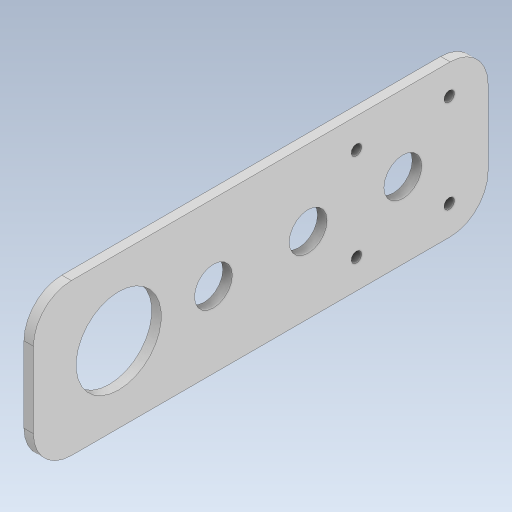
# Autodesk Inventor part: Housing
Saved by Autodesk Inventor 2023 (Build 270158000, 158)
## iProperties
Created: 2023-01-21
Part Number: Housing
Material: Generic
Document SubType Name: Modeling
Designer: Dave
Density: 1 g/cm^3
Appearance: Default
Author: Dave
Autodesk Inventor part; units mm, degrees
ref_plane "YZ Plane" through (0, 0, 0) normal (1, 0, 0) x (0, 1, 0)
ref_plane "XZ Plane" through (0, 0, 0) normal (0, 1, 0) x (-1, 0, 0)
ref_plane "XY Plane" through (0, 0, 0) normal (0, 0, 1) x (1, 0, 0)
sketch "Sketch1" plane through (0, 0, 0) normal (1, 0, 0) x (0, 1, 0)
  line L0 (12.7, 0) -> (38.1, 0)
  line L1 (50.8, -12.7) -> (50.8, -139.7)
  line L2 (38.1, -152.4) -> (12.7, -152.4)
  line L3 (0, -139.7) -> (0, -12.7)
  arc A0 (50.8, -12.7) -> (38.1, 0) centre (38.1, -12.7) ccw
  arc A1 (12.7, 0) -> (0, -12.7) centre (12.7, -12.7) ccw
  arc A2 (0, -139.7) -> (12.7, -152.4) centre (12.7, -139.7) ccw
  arc A3 (38.1, -152.4) -> (50.8, -139.7) centre (38.1, -139.7) ccw
  circle A4 centre (25.4, -28.575) radius 14.2875
  circle A5 centre (25.4, -60.325) radius 6.35
  circle A6 centre (25.4, -92.075) radius 6.35
  circle A7 centre (25.4, -123.825) radius 6.35
  circle A8 centre (25.4, -123.825) radius 22 construction
  circle A9 centre (40.9563, -139.3813) radius 1.75
  circle A10 centre (40.9563, -108.2687) radius 1.75
  circle A11 centre (9.8437, -108.2687) radius 1.75
  circle A12 centre (9.8437, -139.3813) radius 1.75
  line L4 (25.4, -28.575) -> (25.4, -123.825) construction
  point P0 (0, 0)
  point P1 (50.8, -152.4)
  point P2 (50.8, 0)
  point P3 (0, -152.4)
  point P4 (25.4, -152.4)
  point P5 (25.4, -76.2)
  point P6 (0, -76.2)
  dimension "d10" = 44
  dimension "d0" = 50.8
  dimension "d1" = 152.4
  dimension "d2" = 12.7
  dimension "d3" = 28.575
  dimension "d4" = 12.7
  dimension "d5" = 12.7
  dimension "d6" = 12.7
  dimension "d7" = 31.75
  dimension "d8" = 31.75
  dimension "d9" = 31.75
  dimension "d11" = 3.5
  dimension "d14" = 360
  constraints: 12 centre point, 10 end point, 8 point on circle, 8 point on line, 8 tangent, 5 vertical alignment, 3 equal radius, 3 midpoint, 2 parallel, 1 coincident, 1 horizontal, 1 horizontal alignment, 1 perpendicular, 1 vertical, 12 other
  measures "d0" distance of point (50.8, -152.4) point (0, -152.4)
  measures "d1" distance of point (50.8, 0) point (50.8, -152.4)
  measures "d2" radius of A0
  measures "d3" diameter of A4
  measures "d4" diameter of A5
  measures "d5" diameter of A6
  measures "d6" diameter of A7
  measures "d7" distance of L4.start A5.centre
  measures "d8" distance of A6.centre A5.centre
  measures "d9" distance of A7.centre A6.centre
  measures "d11" diameter of A9
extrude "Extrusion1" add sketch "Sketch1" along normal blind 3.175
equation "\"d8\" = d7"
equation "\"d9\" = d7"
body "Solid1"
